Pully_belt calculations v6 (Autodesk Fusion 360 design; units mm, degrees)
Autodesk Fusion 360 part; units mm, degrees
(part 1 of 2)
ref_plane "WorkPlane1" through (0, 0, 0) normal (0, 0, 1) x (1, 0, 0)
sketch "Sketch2" plane through (0, 0, 0) normal (0, 0, 1) x (-1, 0, 0)
  line L0 (0, 0) -> (0, -17.9264) construction
  line L1 (0, 0) -> (0.956, -17.9285) construction
  arc A0 (-0.5778, -17.5255) -> (-0.6732, -17.788) centre (0.4, -18.0295) ccw
  arc A1 (0.6732, -17.788) -> (0.5778, -17.5255) centre (-0.4, -18.0295) ccw
  line L2 (0.6954, -17.9285) -> (-0.6954, -17.9285) construction
  arc A2 (0.5778, -17.5255) -> (-0.5778, -17.5255) centre (0, -17.8233) ccw
  line L3 (0, -17.8233) -> (0, -18.0295) construction
  line L4 (0.4, -18.0295) -> (-0.4, -18.0295) construction
  line L5 (0.8488, -17.9285) -> (0.956, -17.9285)
  line L6 (-0.8488, -17.9285) -> (-0.956, -17.9285)
  arc A3 (0.6732, -17.788) -> (0.8488, -17.9285) centre (0.8488, -17.7485) ccw
  arc A4 (-0.8488, -17.9285) -> (-0.6732, -17.788) centre (-0.8488, -17.7485) ccw
  line L7 (0.956, -17.9285) -> (0.6954, -17.9285) construction
  line L8 (-0.956, -17.9285) -> (-0.6954, -17.9285) construction
  line L9 (0, 0) -> (-0.956, -17.9285) construction
  circle A5 centre (0, 0) radius 17.954 construction
  arc A6 (2.4374, -17.3648) -> (1.2883, -17.4877) centre (1.8945, -17.7224) ccw
  arc A7 (2.5601, -17.6157) -> (2.4374, -17.3648) centre (1.5187, -17.9699) ccw
  arc A8 (2.5601, -17.6157) -> (2.7496, -17.7367) centre (2.7305, -17.5577) ccw
  line L10 (2.7496, -17.7367) -> (2.8563, -17.7253)
  arc A9 (1.0617, -17.9171) -> (1.2214, -17.7588) centre (1.0426, -17.7382) ccw
  arc A10 (1.2883, -17.4877) -> (1.2214, -17.7588) centre (2.3142, -17.8848) ccw
  line L11 (1.0617, -17.9171) -> (0.9551, -17.9285)
  arc A11 (4.2693, -17.0074) -> (3.1399, -17.2517) centre (3.7675, -17.4206) ccw
  arc A12 (4.418, -17.2438) -> (4.2693, -17.0074) centre (3.4202, -17.7066) ccw
  arc A13 (4.418, -17.2438) -> (4.6194, -17.3439) centre (4.5813, -17.168) ccw
  line L12 (4.6194, -17.3439) -> (4.7242, -17.3213)
  arc A14 (2.9602, -17.7028) -> (3.1021, -17.5283) centre (2.9221, -17.5268) ccw
  arc A15 (3.1399, -17.2517) -> (3.1021, -17.5283) centre (4.2021, -17.5375) ccw
  line L13 (2.9602, -17.7028) -> (2.8554, -17.7254)
  arc A16 (6.0529, -16.4572) -> (4.9558, -16.8202) centre (5.5979, -16.9214) ccw
  arc A17 (6.2259, -16.6765) -> (6.0529, -16.4572) centre (5.2829, -17.2428) ccw
  arc A18 (6.2259, -16.6765) -> (6.4367, -16.7547) centre (6.3802, -16.5838) ccw
  line L14 (6.4367, -16.7547) -> (6.5385, -16.721)
  arc A19 (4.8251, -17.2878) -> (4.9477, -17.0993) centre (4.7686, -17.1169) ccw
  arc A20 (4.9558, -16.8202) -> (4.9477, -17.0993) centre (6.0424, -16.9915) ccw
  line L15 (4.8251, -17.2878) -> (4.7233, -17.3215)
  arc A21 (7.7679, -15.7206) -> (6.7156, -16.1981) centre (7.3648, -16.2305) ccw
  arc A22 (7.9632, -15.9202) -> (7.7679, -15.7206) centre (7.0857, -16.5836) ccw
  arc A23 (7.9632, -15.9202) -> (8.1812, -15.9756) centre (8.1068, -15.8117) ccw
  line L16 (8.1812, -15.9756) -> (8.2788, -15.9313)
  arc A24 (6.6353, -16.677) -> (6.7372, -16.4765) centre (6.561, -16.5131) ccw
  arc A25 (6.7156, -16.1981) -> (6.7372, -16.4765) centre (7.8143, -16.253) ccw
  line L17 (6.6353, -16.677) -> (6.5377, -16.7213)
  arc A26 (9.3949, -14.8059) -> (8.3993, -15.3925) centre (9.0483, -15.3558) ccw
  arc A27 (9.6103, -14.9836) -> (9.3949, -14.8059) centre (8.8083, -15.7364) ccw
  arc A28 (9.6103, -14.9836) -> (9.8329, -15.0155) centre (9.7416, -14.8604) ccw
  line L18 (9.8329, -15.0155) -> (9.9253, -14.961)
  arc A29 (8.3704, -15.8772) -> (8.4504, -15.6671) centre (8.279, -15.7222) ccw
  arc A30 (8.3993, -15.3925) -> (8.4504, -15.6671) centre (9.4976, -15.3303) ccw
  line L19 (8.3704, -15.8772) -> (8.278, -15.9317)
  arc A31 (10.9155, -13.7234) -> (9.9879, -14.4125) centre (10.6293, -14.307) ccw
  arc A32 (11.1485, -13.8772) -> (10.9155, -13.7234) centre (10.4311, -14.711) ccw
  arc A33 (11.1485, -13.8772) -> (11.3733, -13.8852) centre (11.2659, -13.7407) ccw
  line L20 (11.3733, -13.8852) -> (11.4594, -13.8213)
  arc A34 (10.0106, -14.8976) -> (10.0678, -14.6801) centre (9.9033, -14.7531) ccw
  arc A35 (9.9879, -14.4125) -> (10.0678, -14.6801) centre (11.0733, -14.2339) ccw
  line L21 (10.0106, -14.8976) -> (9.9246, -14.9615)
  arc A36 (12.3123, -12.4854) -> (11.4633, -13.2692) centre (12.0898, -13.0961) ccw
  arc A37 (12.5604, -12.6135) -> (12.3123, -12.4854) centre (11.9357, -13.5189) ccw
  arc A38 (12.5604, -12.6135) -> (12.7848, -12.5977) centre (12.6627, -12.4654) ccw
  line L22 (12.7848, -12.5977) -> (12.8635, -12.5249)
  arc A39 (11.5374, -13.7491) -> (11.5712, -13.5268) centre (11.4153, -13.6169) ccw
  arc A40 (11.4633, -13.2692) -> (11.5712, -13.5268) centre (12.5235, -12.9763) ccw
  line L23 (11.5374, -13.7491) -> (11.4587, -13.8219)
  arc A41 (13.5697, -11.106) -> (12.8087, -11.9756) centre (13.4133, -11.7369) ccw
  arc A42 (13.83, -11.207) -> (13.5697, -11.106) centre (13.3051, -12.1736) ccw
  arc A43 (13.83, -11.207) -> (14.0514, -11.1673) centre (13.9159, -11.0488) ccw
  line L24 (14.0514, -11.1673) -> (14.122, -11.0867)
  arc A44 (12.9335, -12.4449) -> (12.9434, -12.2202) centre (12.7981, -12.3263) ccw
  arc A45 (12.8087, -11.9756) -> (12.9434, -12.2202) centre (13.8319, -11.5716) ccw
  line L25 (12.9335, -12.4449) -> (12.8629, -12.5256)
  arc A46 (14.6733, -9.6007) -> (14.0091, -10.5463) centre (14.5849, -10.2446) ccw
  arc A47 (14.9429, -9.6735) -> (14.6733, -9.6007) centre (14.5237, -10.6904) ccw
  arc A48 (14.9429, -9.6735) -> (15.1588, -9.6105) centre (15.0115, -9.507) ccw
  line L26 (15.1588, -9.6105) -> (15.2204, -9.5228)
  arc A49 (14.1831, -10.9996) -> (14.169, -10.7752) centre (14.0358, -10.8962) ccw
  arc A50 (14.0091, -10.5463) -> (14.169, -10.7752) centre (14.9835, -10.0358) ccw
  line L27 (14.1831, -10.9996) -> (14.1214, -11.0874)
  arc A51 (15.6107, -7.9866) -> (15.0507, -8.9974) centre (15.5912, -8.6363) ccw
  arc A52 (15.8865, -8.0303) -> (15.6107, -7.9866) centre (15.5777, -9.0861) ccw
  arc A53 (15.8865, -8.0303) -> (16.0944, -7.9448) centre (15.937, -7.8576) ccw
  line L28 (16.0944, -7.9448) -> (16.1464, -7.851)
  arc A54 (15.2719, -9.4297) -> (15.2341, -9.208) centre (15.1144, -9.3425) ccw
  arc A55 (15.0507, -8.9974) -> (15.2341, -9.208) centre (15.9653, -8.3863) ccw
  line L29 (15.2719, -9.4297) -> (15.2199, -9.5235)
  arc A56 (16.3712, -6.282) -> (15.9218, -7.3467) centre (16.4208, -6.9301) ccw
  arc A57 (16.65, -6.2962) -> (16.3712, -6.282) centre (16.4552, -7.3788) ccw
  arc A58 (16.65, -6.2962) -> (16.8477, -6.189) centre (16.6819, -6.1191) ccw
  line L30 (16.8477, -6.189) -> (16.8894, -6.0903)
  arc A59 (16.1877, -7.753) -> (16.1266, -7.5366) centre (16.0219, -7.683) ccw
  arc A60 (15.9218, -7.3467) -> (16.1266, -7.5366) centre (16.7663, -6.6418) ccw
  line L31 (16.1877, -7.753) -> (16.146, -7.8518)
  arc A61 (16.9461, -4.5063) -> (16.6125, -5.6127) centre (17.0644, -5.1455) ccw
  arc A62 (17.225, -4.4907) -> (16.9461, -4.5063) centre (17.1463, -5.5879) ccw
  arc A63 (17.225, -4.4907) -> (17.4102, -4.3632) centre (17.2378, -4.3112) ccw
  line L32 (17.4102, -4.3632) -> (17.4411, -4.2605)
  arc A64 (16.9201, -5.9884) -> (16.8363, -5.7798) centre (16.7478, -5.9365) ccw
  arc A65 (16.6125, -5.6127) -> (16.8363, -5.7798) centre (17.3773, -4.822) ccw
  line L33 (16.9201, -5.9884) -> (16.8891, -6.0911)
  arc A66 (17.3291, -2.6795) -> (17.115, -3.8151) centre (17.5147, -3.3025) ccw
  arc A67 (17.6047, -2.6344) -> (17.3291, -2.6795) centre (17.6432, -3.7337) ccw
  arc A68 (17.6047, -2.6344) -> (17.7753, -2.4879) centre (17.5984, -2.4545) ccw
  line L34 (17.7753, -2.4879) -> (17.7952, -2.3825)
  arc A69 (17.4608, -4.156) -> (17.3553, -3.9574) centre (17.2839, -4.1227) ccw
  arc A70 (17.115, -3.8151) -> (17.3553, -3.9574) centre (17.7914, -2.9476) ccw
  line L35 (17.4608, -4.156) -> (17.4409, -4.2614)
  arc A71 (17.5158, -0.8224) -> (17.4236, -1.9742) centre (17.7665, -1.4221) ccw
  arc A72 (17.785, -0.7482) -> (17.5158, -0.8224) centre (17.9401, -1.8372) ccw
  arc A73 (17.785, -0.7482) -> (17.939, -0.5844) centre (17.7596, -0.57) ccw
  line L36 (17.939, -0.5844) -> (17.9476, -0.4775)
  arc A74 (17.8036, -2.2765) -> (17.6776, -2.0903) centre (17.6242, -2.2622) ccw
  arc A75 (17.4236, -1.9742) -> (17.6776, -2.0903) centre (18.0039, -1.0398) ccw
  line L37 (17.8036, -2.2765) -> (17.795, -2.3834)
  arc A76 (17.504, 1.0441) -> (17.5347, -0.111) centre (17.817, 0.4745) ccw
  arc A77 (17.7638, 1.1465) -> (17.504, 1.0441) centre (18.0337, 0.0801) ccw
  arc A78 (17.7638, 1.1465) -> (17.8995, 1.3257) centre (17.7196, 1.3209) ccw
  line L38 (17.8995, 1.3257) -> (17.8967, 1.4329)
  arc A79 (17.9447, -0.3712) -> (17.7996, -0.1994) centre (17.7648, -0.376) ccw
  arc A80 (17.5347, -0.111) -> (17.7996, -0.1994) centre (18.0124, 0.8798) ccw
  line L39 (17.9447, -0.3712) -> (17.9476, -0.4784)
  arc A81 (17.2938, 2.8988) -> (17.4472, 1.7534) centre (17.6656, 2.3656) ccw
  arc A82 (17.5413, 3.0281) -> (17.2938, 2.8988) centre (17.9231, 1.9965) ccw
  arc A83 (17.5413, 3.0281) -> (17.6572, 3.2208) centre (17.4788, 3.1969) ccw
  line L40 (17.6572, 3.2208) -> (17.643, 3.3271)
  arc A84 (17.8825, 1.5383) -> (17.72, 1.6937) centre (17.7041, 1.5144) ccw
  arc A85 (17.4472, 1.7534) -> (17.72, 1.6937) centre (17.8169, 2.7894) ccw
  line L41 (17.8825, 1.5383) -> (17.8967, 1.432)
  arc A86 (16.8877, 4.7206) -> (17.162, 3.598) centre (17.3141, 4.23) ccw
  arc A87 (17.12, 4.8755) -> (16.8877, 4.7206) centre (17.6093, 3.8903) ccw
  arc A88 (17.12, 4.8755) -> (17.2148, 5.0794) centre (17.04, 5.0367) ccw
  line L42 (17.2148, 5.0794) -> (17.1894, 5.1836)
  arc A89 (17.6177, 3.4304) -> (17.4396, 3.5676) centre (17.4428, 3.3877) ccw
  arc A90 (17.162, 3.598) -> (17.4396, 3.5676) centre (17.4194, 4.6674) ccw
  line L43 (17.6177, 3.4304) -> (17.6431, 3.3262)
  arc A91 (16.2903, 6.4889) -> (16.6823, 5.4018) centre (16.7664, 6.0464) ccw
  arc A92 (16.5048, 6.6676) -> (16.2903, 6.4889) centre (17.096, 5.74) ccw
  arc A93 (16.5048, 6.6676) -> (16.5774, 6.8805) centre (16.4081, 6.8194) ccw
  line L44 (16.5774, 6.8805) -> (16.541, 6.9813)
  arc A94 (17.1533, 5.2836) -> (16.9615, 5.4011) centre (16.9839, 5.2225) ccw
  arc A95 (16.6823, 5.4018) -> (16.9615, 5.4011) centre (16.8246, 6.4926) ccw
  line L45 (17.1533, 5.2836) -> (17.1896, 5.1827)
  arc A96 (15.5083, 8.1837) -> (16.0136, 7.1444) centre (16.0287, 7.7943) ccw
  arc A97 (15.7026, 8.3842) -> (15.5083, 8.1837) centre (16.3891, 7.5247) ccw
  arc A98 (15.7026, 8.3842) -> (15.7521, 8.6036) centre (15.5902, 8.5249) ccw
  line L46 (15.7521, 8.6036) -> (15.7052, 8.7)
  arc A99 (16.4945, 7.0769) -> (16.2913, 7.1734) centre (16.3326, 6.9982) ccw
  arc A100 (16.0136, 7.1444) -> (16.2913, 7.1734) centre (16.0392, 8.2441) ccw
  line L47 (16.4945, 7.0769) -> (16.5414, 6.9805)
  arc A101 (14.5505, 9.7857) -> (15.1635, 8.8061) centre (15.1094, 9.4539) ccw
  arc A102 (14.7224, 10.0058) -> (14.5505, 9.7857) centre (15.4964, 9.2241) ccw
  arc A103 (14.7224, 10.0058) -> (14.7484, 10.2292) centre (14.5958, 10.1337) ccw
  line L48 (14.7484, 10.2292) -> (14.6915, 10.3201)
  arc A104 (15.6488, 8.7901) -> (15.4366, 8.8645) centre (15.4962, 8.6946) ccw
  arc A105 (15.1635, 8.8061) -> (15.4366, 8.8645) centre (15.072, 9.9023) ccw
  line L49 (15.6488, 8.7901) -> (15.7057, 8.6992)
  arc A106 (13.428, 11.2769) -> (14.1415, 10.368) centre (14.019, 11.0063) ccw
  arc A107 (13.5755, 11.514) -> (13.428, 11.2769) centre (14.4281, 10.819) ccw
  arc A108 (13.5755, 11.514) -> (13.5775, 11.7389) centre (13.436, 11.6277) ccw
  line L50 (13.5775, 11.7389) -> (13.5113, 11.8232)
  arc A109 (14.6258, 10.4037) -> (14.4069, 10.455) centre (14.4842, 10.2925) ccw
  arc A110 (14.1415, 10.368) -> (14.4069, 10.455) centre (13.9341, 11.4483) ccw
  line L51 (14.6258, 10.4037) -> (14.692, 10.3193)
  arc A111 (12.1532, 12.6403) -> (12.9594, 11.8124) centre (12.7696, 12.4341) ccw
  arc A112 (12.2747, 12.8918) -> (12.1532, 12.6403) centre (13.1964, 12.2914) ccw
  arc A113 (12.2747, 12.8918) -> (12.2528, 13.1156) centre (12.1239, 12.99) ccw
  line L52 (12.2528, 13.1156) -> (12.178, 13.1924)
  arc A114 (13.4371, 11.8994) -> (13.214, 11.9272) centre (13.3082, 11.7738) ccw
  arc A115 (12.9594, 11.8124) -> (13.214, 11.9272) centre (12.6383, 12.8645) ccw
  line L53 (13.4371, 11.8994) -> (13.5119, 11.8225)
  arc A116 (10.7408, 13.8605) -> (11.6304, 13.123) centre (11.3756, 13.721) ccw
  arc A117 (10.8349, 14.1234) -> (10.7408, 13.8605) centre (11.8151, 13.6244) ccw
  arc A118 (10.8349, 14.1234) -> (10.7893, 14.3437) centre (10.6744, 14.2051) ccw
  line L54 (10.7893, 14.3437) -> (10.7068, 14.4121)
  arc A119 (12.0962, 13.2602) -> (11.8713, 13.2642) centre (11.9813, 13.1217) ccw
  arc A120 (11.6304, 13.123) -> (11.8713, 13.2642) centre (11.1993, 14.135) ccw
  line L55 (12.0962, 13.2602) -> (12.1787, 13.1918)
  arc A121 (9.2067, 14.9237) -> (10.1696, 14.2849) centre (9.8527, 14.8524) ccw
  arc A122 (9.2722, 15.1951) -> (9.2067, 14.9237) centre (10.3, 14.8031) ccw
  arc A123 (9.2722, 15.1951) -> (9.2036, 15.4093) centre (9.1041, 15.2593) ccw
  line L56 (9.2036, 15.4093) -> (9.1142, 15.4685)
  arc A124 (10.6182, 14.4708) -> (10.3942, 14.4509) centre (10.5187, 14.3209) ccw
  arc A125 (10.1696, 14.2849) -> (10.3942, 14.4509) centre (9.6334, 15.2453) ccw
  line L57 (10.6182, 14.4708) -> (10.7075, 14.4116)
  arc A126 (7.5682, 15.8177) -> (8.5936, 15.2849) centre (8.2182, 15.8156) ccw
  arc A127 (7.6046, 16.0946) -> (7.5682, 15.8177) centre (8.6682, 15.8141) ccw
  arc A128 (7.6046, 16.0946) -> (7.5135, 16.3002) centre (7.4305, 16.1405) ccw
  line L58 (7.5135, 16.3002) -> (7.4184, 16.3497)
  arc A129 (9.0199, 15.5175) -> (8.7992, 15.4738) centre (8.9369, 15.3578) ccw
  arc A130 (8.5936, 15.2849) -> (8.7992, 15.4738) centre (7.9583, 16.1829) ccw
  line L59 (9.0199, 15.5175) -> (9.115, 15.4681)
  arc A131 (5.844, 16.5326) -> (6.9202, 16.1118) centre (6.4906, 16.5995) ccw
  arc A132 (5.8507, 16.8117) -> (5.844, 16.5326) centre (6.9382, 16.6458) ccw
  arc A133 (5.8507, 16.8117) -> (5.7384, 17.0065) centre (5.6728, 16.8389) ccw
  line L60 (5.7384, 17.0065) -> (5.6385, 17.0456)
  arc A134 (7.3193, 16.3884) -> (7.1046, 16.3215) centre (7.2538, 16.2207) ccw
  arc A135 (6.9202, 16.1118) -> (7.1046, 16.3215) centre (6.1931, 16.9372) ccw
  line L61 (7.3193, 16.3884) -> (7.4192, 16.3493)
  arc A136 (4.0536, 17.0601) -> (5.1684, 16.7561) centre (4.6894, 17.1954) ccw
  arc A137 (4.0306, 17.3384) -> (4.0536, 17.0601) centre (5.1295, 17.289) ccw
  arc A138 (4.0306, 17.3384) -> (3.8982, 17.5201) centre (3.8508, 17.3465) ccw
  line L62 (3.8982, 17.5201) -> (3.7947, 17.5483)
  arc A139 (5.5359, 17.0735) -> (5.3295, 16.9842) centre (5.4885, 16.8998) ccw
  arc A140 (5.1684, 16.7561) -> (5.3295, 16.9842) centre (4.3577, 17.4995) ccw
  line L63 (5.5359, 17.0735) -> (5.6393, 17.0453)
  arc A141 (2.2173, 17.3943) -> (3.3581, 17.2105) centre (2.835, 17.5964) ccw
  arc A142 (2.1648, 17.6686) -> (2.2173, 17.3943) centre (3.2627, 17.7363) ccw
  arc A143 (2.1648, 17.6686) -> (2.0138, 17.8352) centre (1.9852, 17.6575) ccw
  line L64 (2.0138, 17.8352) -> (1.9079, 17.8523)
  arc A144 (3.6897, 17.5652) -> (3.494, 17.4544) centre (3.6611, 17.3875) ccw
  arc A145 (3.3581, 17.2105) -> (3.494, 17.4544) centre (2.4729, 17.8636) ccw
  line L65 (3.6897, 17.5652) -> (3.7956, 17.5482)
  arc A146 (0.3558, 17.5315) -> (1.5097, 17.47) centre (0.9486, 17.7981) ccw
  arc A147 (0.2745, 17.7986) -> (0.3558, 17.5315) centre (1.359, 17.9826) ccw
  arc A148 (0.2745, 17.7986) -> (0.1066, 17.9482) centre (0.097, 17.7685) ccw
  line L66 (0.1066, 17.9482) -> (-0.0005, 17.954)
  arc A149 (1.8018, 17.8579) -> (1.6189, 17.727) centre (1.7922, 17.6782) ccw
  arc A150 (1.5097, 17.47) -> (1.6189, 17.727) centre (0.5601, 18.0252) ccw
  line L67 (1.8018, 17.8579) -> (1.9088, 17.8522)
  arc A151 (-1.5097, 17.47) -> (-0.3558, 17.5315) centre (-0.9486, 17.7981) ccw
  arc A152 (-1.6189, 17.727) -> (-1.5097, 17.47) centre (-0.5601, 18.0252) ccw
  arc A153 (-1.6189, 17.727) -> (-1.8018, 17.8579) centre (-1.7922, 17.6782) ccw
  line L68 (-1.8018, 17.8579) -> (-1.9088, 17.8522)
  arc A154 (-0.1066, 17.9482) -> (-0.2745, 17.7986) centre (-0.097, 17.7685) ccw
  arc A155 (-0.3558, 17.5315) -> (-0.2745, 17.7986) centre (-1.359, 17.9826) ccw
  line L69 (-0.1066, 17.9482) -> (0.0005, 17.954)
  arc A156 (-3.3581, 17.2105) -> (-2.2173, 17.3943) centre (-2.835, 17.5964) ccw
  arc A157 (-3.494, 17.4544) -> (-3.3581, 17.2105) centre (-2.4729, 17.8636) ccw
  arc A158 (-3.494, 17.4544) -> (-3.6897, 17.5652) centre (-3.6611, 17.3875) ccw
  line L70 (-3.6897, 17.5652) -> (-3.7956, 17.5482)
  arc A159 (-2.0138, 17.8352) -> (-2.1648, 17.6686) centre (-1.9852, 17.6575) ccw
  arc A160 (-2.2173, 17.3943) -> (-2.1648, 17.6686) centre (-3.2627, 17.7363) ccw
  line L71 (-2.0138, 17.8352) -> (-1.9079, 17.8523)
  arc A161 (-5.1684, 16.7561) -> (-4.0536, 17.0601) centre (-4.6894, 17.1954) ccw
  arc A162 (-5.3295, 16.9842) -> (-5.1684, 16.7561) centre (-4.3577, 17.4995) ccw
  arc A163 (-5.3295, 16.9842) -> (-5.5359, 17.0735) centre (-5.4885, 16.8998) ccw
  line L72 (-5.5359, 17.0735) -> (-5.6393, 17.0453)
  arc A164 (-3.8982, 17.5201) -> (-4.0306, 17.3384) centre (-3.8508, 17.3465) ccw
  arc A165 (-4.0536, 17.0601) -> (-4.0306, 17.3384) centre (-5.1295, 17.289) ccw
  line L73 (-3.8982, 17.5201) -> (-3.7947, 17.5483)
  arc A166 (-6.9202, 16.1118) -> (-5.844, 16.5326) centre (-6.4906, 16.5995) ccw
  arc A167 (-7.1046, 16.3215) -> (-6.9202, 16.1118) centre (-6.1931, 16.9372) ccw
  arc A168 (-7.1046, 16.3215) -> (-7.3193, 16.3884) centre (-7.2538, 16.2207) ccw
  line L74 (-7.3193, 16.3884) -> (-7.4192, 16.3493)
  arc A169 (-5.7384, 17.0065) -> (-5.8507, 16.8117) centre (-5.6728, 16.8389) ccw
  arc A170 (-5.844, 16.5326) -> (-5.8507, 16.8117) centre (-6.9382, 16.6458) ccw
  line L75 (-5.7384, 17.0065) -> (-5.6385, 17.0456)
  arc A171 (-8.5936, 15.2849) -> (-7.5682, 15.8177) centre (-8.2182, 15.8156) ccw
  arc A172 (-8.7992, 15.4738) -> (-8.5936, 15.2849) centre (-7.9583, 16.1829) ccw
  arc A173 (-8.7992, 15.4738) -> (-9.0199, 15.5175) centre (-8.9369, 15.3578) ccw
  line L76 (-9.0199, 15.5175) -> (-9.115, 15.4681)
  arc A174 (-7.5135, 16.3002) -> (-7.6046, 16.0946) centre (-7.4305, 16.1405) ccw
  arc A175 (-7.5682, 15.8177) -> (-7.6046, 16.0946) centre (-8.6682, 15.8141) ccw
  line L77 (-7.5135, 16.3002) -> (-7.4184, 16.3497)
  arc A176 (-10.1696, 14.2849) -> (-9.2067, 14.9237) centre (-9.8527, 14.8524) ccw
  arc A177 (-10.3942, 14.4509) -> (-10.1696, 14.2849) centre (-9.6334, 15.2453) ccw
  arc A178 (-10.3942, 14.4509) -> (-10.6182, 14.4708) centre (-10.5187, 14.3209) ccw
  line L78 (-10.6182, 14.4708) -> (-10.7075, 14.4116)
  arc A179 (-9.2036, 15.4093) -> (-9.2722, 15.1951) centre (-9.1041, 15.2593) ccw
  arc A180 (-9.2067, 14.9237) -> (-9.2722, 15.1951) centre (-10.3, 14.8031) ccw
  line L79 (-9.2036, 15.4093) -> (-9.1142, 15.4685)
  arc A181 (-11.6304, 13.123) -> (-10.7408, 13.8605) centre (-11.3756, 13.721) ccw
  arc A182 (-11.8713, 13.2642) -> (-11.6304, 13.123) centre (-11.1993, 14.135) ccw
  arc A183 (-11.8713, 13.2642) -> (-12.0962, 13.2602) centre (-11.9813, 13.1217) ccw
  line L80 (-12.0962, 13.2602) -> (-12.1787, 13.1918)
  arc A184 (-10.7893, 14.3437) -> (-10.8349, 14.1234) centre (-10.6744, 14.2051) ccw
  arc A185 (-10.7408, 13.8605) -> (-10.8349, 14.1234) centre (-11.8151, 13.6244) ccw
  line L81 (-10.7893, 14.3437) -> (-10.7068, 14.4121)
  arc A186 (-12.9594, 11.8124) -> (-12.1532, 12.6403) centre (-12.7696, 12.4341) ccw
  arc A187 (-13.214, 11.9272) -> (-12.9594, 11.8124) centre (-12.6383, 12.8645) ccw
  arc A188 (-13.214, 11.9272) -> (-13.4371, 11.8994) centre (-13.3082, 11.7738) ccw
  line L82 (-13.4371, 11.8994) -> (-13.5119, 11.8225)
  arc A189 (-12.2528, 13.1156) -> (-12.2747, 12.8918) centre (-12.1239, 12.99) ccw
  arc A190 (-12.1532, 12.6403) -> (-12.2747, 12.8918) centre (-13.1964, 12.2914) ccw
  line L83 (-12.2528, 13.1156) -> (-12.178, 13.1924)
  arc A191 (-14.1415, 10.368) -> (-13.428, 11.2769) centre (-14.019, 11.0063) ccw
  arc A192 (-14.4069, 10.455) -> (-14.1415, 10.368) centre (-13.9341, 11.4483) ccw
  arc A193 (-14.4069, 10.455) -> (-14.6258, 10.4037) centre (-14.4842, 10.2925) ccw
  line L84 (-14.6258, 10.4037) -> (-14.692, 10.3193)
  arc A194 (-13.5775, 11.7389) -> (-13.5755, 11.514) centre (-13.436, 11.6277) ccw
  arc A195 (-13.428, 11.2769) -> (-13.5755, 11.514) centre (-14.4281, 10.819) ccw
  line L85 (-13.5775, 11.7389) -> (-13.5113, 11.8232)
  arc A196 (-15.1635, 8.8061) -> (-14.5505, 9.7857) centre (-15.1094, 9.4539) ccw
  arc A197 (-15.4366, 8.8645) -> (-15.1635, 8.8061) centre (-15.072, 9.9023) ccw
  arc A198 (-15.4366, 8.8645) -> (-15.6488, 8.7901) centre (-15.4962, 8.6946) ccw
  line L86 (-15.6488, 8.7901) -> (-15.7057, 8.6992)
  arc A199 (-14.7484, 10.2292) -> (-14.7224, 10.0058) centre (-14.5958, 10.1337) ccw
  arc A200 (-14.5505, 9.7857) -> (-14.7224, 10.0058) centre (-15.4964, 9.2241) ccw
  line L87 (-14.7484, 10.2292) -> (-14.6915, 10.3201)
  arc A201 (-16.0136, 7.1444) -> (-15.5083, 8.1837) centre (-16.0287, 7.7943) ccw
  arc A202 (-16.2913, 7.1734) -> (-16.0136, 7.1444) centre (-16.0392, 8.2441) ccw
  arc A203 (-16.2913, 7.1734) -> (-16.4945, 7.0769) centre (-16.3326, 6.9982) ccw
  line L88 (-16.4945, 7.0769) -> (-16.5414, 6.9805)
  arc A204 (-15.7521, 8.6036) -> (-15.7026, 8.3842) centre (-15.5902, 8.5249) ccw
  arc A205 (-15.5083, 8.1837) -> (-15.7026, 8.3842) centre (-16.3891, 7.5247) ccw
  line L89 (-15.7521, 8.6036) -> (-15.7052, 8.7)
  arc A206 (-16.6823, 5.4018) -> (-16.2903, 6.4889) centre (-16.7664, 6.0464) ccw
  arc A207 (-16.9615, 5.4011) -> (-16.6823, 5.4018) centre (-16.8246, 6.4926) ccw
  arc A208 (-16.9615, 5.4011) -> (-17.1533, 5.2836) centre (-16.9839, 5.2225) ccw
  line L90 (-17.1533, 5.2836) -> (-17.1896, 5.1827)
  arc A209 (-16.5774, 6.8805) -> (-16.5048, 6.6676) centre (-16.4081, 6.8194) ccw
  arc A210 (-16.2903, 6.4889) -> (-16.5048, 6.6676) centre (-17.096, 5.74) ccw
  line L91 (-16.5774, 6.8805) -> (-16.541, 6.9813)
  arc A211 (-17.162, 3.598) -> (-16.8877, 4.7206) centre (-17.3141, 4.23) ccw
  arc A212 (-17.4396, 3.5676) -> (-17.162, 3.598) centre (-17.4194, 4.6674) ccw
  arc A213 (-17.4396, 3.5676) -> (-17.6177, 3.4304) centre (-17.4428, 3.3877) ccw
  line L92 (-17.6177, 3.4304) -> (-17.6431, 3.3262)
  arc A214 (-17.2148, 5.0794) -> (-17.12, 4.8755) centre (-17.04, 5.0367) ccw
  arc A215 (-16.8877, 4.7206) -> (-17.12, 4.8755) centre (-17.6093, 3.8903) ccw
  line L93 (-17.2148, 5.0794) -> (-17.1894, 5.1836)
  arc A216 (-17.4472, 1.7534) -> (-17.2938, 2.8988) centre (-17.6656, 2.3656) ccw
  arc A217 (-17.72, 1.6937) -> (-17.4472, 1.7534) centre (-17.8169, 2.7894) ccw
  arc A218 (-17.72, 1.6937) -> (-17.8825, 1.5383) centre (-17.7041, 1.5144) ccw
  line L94 (-17.8825, 1.5383) -> (-17.8967, 1.432)
  arc A219 (-17.6572, 3.2208) -> (-17.5413, 3.0281) centre (-17.4788, 3.1969) ccw
  arc A220 (-17.2938, 2.8988) -> (-17.5413, 3.0281) centre (-17.9231, 1.9965) ccw
  line L95 (-17.6572, 3.2208) -> (-17.643, 3.3271)
  arc A221 (-17.5347, -0.111) -> (-17.504, 1.0441) centre (-17.817, 0.4745) ccw
  arc A222 (-17.7996, -0.1994) -> (-17.5347, -0.111) centre (-18.0124, 0.8798) ccw
  arc A223 (-17.7996, -0.1994) -> (-17.9447, -0.3712) centre (-17.7648, -0.376) ccw
  line L96 (-17.9447, -0.3712) -> (-17.9476, -0.4784)
  arc A224 (-17.8995, 1.3257) -> (-17.7638, 1.1465) centre (-17.7196, 1.3209) ccw
  arc A225 (-17.504, 1.0441) -> (-17.7638, 1.1465) centre (-18.0337, 0.0801) ccw
  line L97 (-17.8995, 1.3257) -> (-17.8967, 1.4329)
  arc A226 (-17.4236, -1.9742) -> (-17.5158, -0.8224) centre (-17.7665, -1.4221) ccw
  arc A227 (-17.6776, -2.0903) -> (-17.4236, -1.9742) centre (-18.0039, -1.0398) ccw
  arc A228 (-17.6776, -2.0903) -> (-17.8036, -2.2765) centre (-17.6242, -2.2622) ccw
  line L98 (-17.8036, -2.2765) -> (-17.795, -2.3834)
  arc A229 (-17.939, -0.5844) -> (-17.785, -0.7482) centre (-17.7596, -0.57) ccw
  arc A230 (-17.5158, -0.8224) -> (-17.785, -0.7482) centre (-17.9401, -1.8372) ccw
  line L99 (-17.939, -0.5844) -> (-17.9476, -0.4775)
  arc A231 (-17.115, -3.8151) -> (-17.3291, -2.6795) centre (-17.5147, -3.3025) ccw
  arc A232 (-17.3553, -3.9574) -> (-17.115, -3.8151) centre (-17.7914, -2.9476) ccw
  arc A233 (-17.3553, -3.9574) -> (-17.4608, -4.156) centre (-17.2839, -4.1227) ccw
  line L100 (-17.4608, -4.156) -> (-17.4409, -4.2614)
  arc A234 (-17.7753, -2.4879) -> (-17.6047, -2.6344) centre (-17.5984, -2.4545) ccw
  arc A235 (-17.3291, -2.6795) -> (-17.6047, -2.6344) centre (-17.6432, -3.7337) ccw
  line L101 (-17.7753, -2.4879) -> (-17.7952, -2.3825)
  arc A236 (-16.6125, -5.6127) -> (-16.9461, -4.5063) centre (-17.0644, -5.1455) ccw
  arc A237 (-16.8363, -5.7798) -> (-16.6125, -5.6127) centre (-17.3773, -4.822) ccw
  arc A238 (-16.8363, -5.7798) -> (-16.9201, -5.9884) centre (-16.7478, -5.9365) ccw
  line L102 (-16.9201, -5.9884) -> (-16.8891, -6.0911)
  arc A239 (-17.4102, -4.3632) -> (-17.225, -4.4907) centre (-17.2378, -4.3112) ccw
  arc A240 (-16.9461, -4.5063) -> (-17.225, -4.4907) centre (-17.1463, -5.5879) ccw
  line L103 (-17.4102, -4.3632) -> (-17.4411, -4.2605)
  arc A241 (-15.9218, -7.3467) -> (-16.3712, -6.282) centre (-16.4208, -6.9301) ccw
  arc A242 (-16.1266, -7.5366) -> (-15.9218, -7.3467) centre (-16.7663, -6.6418) ccw
  arc A243 (-16.1266, -7.5366) -> (-16.1877, -7.753) centre (-16.0219, -7.683) ccw
  line L104 (-16.1877, -7.753) -> (-16.146, -7.8518)
  arc A244 (-16.8477, -6.189) -> (-16.65, -6.2962) centre (-16.6819, -6.1191) ccw
  arc A245 (-16.3712, -6.282) -> (-16.65, -6.2962) centre (-16.4552, -7.3788) ccw
  line L105 (-16.8477, -6.189) -> (-16.8894, -6.0903)
  arc A246 (-15.0507, -8.9974) -> (-15.6107, -7.9866) centre (-15.5912, -8.6363) ccw
  arc A247 (-15.2341, -9.208) -> (-15.0507, -8.9974) centre (-15.9653, -8.3863) ccw
  arc A248 (-15.2341, -9.208) -> (-15.2719, -9.4297) centre (-15.1144, -9.3425) ccw
  line L106 (-15.2719, -9.4297) -> (-15.2199, -9.5235)
  arc A249 (-16.0944, -7.9448) -> (-15.8865, -8.0303) centre (-15.937, -7.8576) ccw
  arc A250 (-15.6107, -7.9866) -> (-15.8865, -8.0303) centre (-15.5777, -9.0861) ccw
  line L107 (-16.0944, -7.9448) -> (-16.1464, -7.851)
  arc A251 (-14.0091, -10.5463) -> (-14.6733, -9.6007) centre (-14.5849, -10.2446) ccw
  arc A252 (-14.169, -10.7752) -> (-14.0091, -10.5463) centre (-14.9835, -10.0358) ccw
  arc A253 (-14.169, -10.7752) -> (-14.1831, -10.9996) centre (-14.0358, -10.8962) ccw
  line L108 (-14.1831, -10.9996) -> (-14.1214, -11.0874)
  arc A254 (-15.1588, -9.6105) -> (-14.9429, -9.6735) centre (-15.0115, -9.507) ccw
  arc A255 (-14.6733, -9.6007) -> (-14.9429, -9.6735) centre (-14.5237, -10.6904) ccw
  line L109 (-15.1588, -9.6105) -> (-15.2204, -9.5228)
  arc A256 (-12.8087, -11.9756) -> (-13.5697, -11.106) centre (-13.4133, -11.7369) ccw
  arc A257 (-12.9434, -12.2202) -> (-12.8087, -11.9756) centre (-13.8319, -11.5716) ccw
  arc A258 (-12.9434, -12.2202) -> (-12.9335, -12.4449) centre (-12.7981, -12.3263) ccw
  line L110 (-12.9335, -12.4449) -> (-12.8629, -12.5256)
  arc A259 (-14.0514, -11.1673) -> (-13.83, -11.207) centre (-13.9159, -11.0488) ccw
  arc A260 (-13.5697, -11.106) -> (-13.83, -11.207) centre (-13.3051, -12.1736) ccw
  line L111 (-14.0514, -11.1673) -> (-14.122, -11.0867)
  arc A261 (-11.4633, -13.2692) -> (-12.3123, -12.4854) centre (-12.0898, -13.0961) ccw
  arc A262 (-11.5712, -13.5268) -> (-11.4633, -13.2692) centre (-12.5235, -12.9763) ccw
  arc A263 (-11.5712, -13.5268) -> (-11.5374, -13.7491) centre (-11.4153, -13.6169) ccw
  line L112 (-11.5374, -13.7491) -> (-11.4587, -13.8219)
  arc A264 (-12.7848, -12.5976) -> (-12.5604, -12.6135) centre (-12.6627, -12.4654) ccw
  arc A265 (-12.3123, -12.4854) -> (-12.5604, -12.6135) centre (-11.9357, -13.5189) ccw
  line L113 (-12.7848, -12.5976) -> (-12.8635, -12.5249)
  arc A266 (-9.9879, -14.4125) -> (-10.9155, -13.7234) centre (-10.6293, -14.307) ccw
  arc A267 (-10.0678, -14.6801) -> (-9.9879, -14.4125) centre (-11.0733, -14.2339) ccw
  arc A268 (-10.0678, -14.6801) -> (-10.0106, -14.8976) centre (-9.9033, -14.7531) ccw
  line L114 (-10.0106, -14.8976) -> (-9.9246, -14.9615)
  arc A269 (-11.3733, -13.8852) -> (-11.1485, -13.8772) centre (-11.2659, -13.7407) ccw
  arc A270 (-10.9155, -13.7234) -> (-11.1485, -13.8772) centre (-10.4311, -14.711) ccw
  line L115 (-11.3733, -13.8852) -> (-11.4594, -13.8213)
  arc A271 (-8.3993, -15.3925) -> (-9.3949, -14.8059) centre (-9.0483, -15.3558) ccw
  arc A272 (-8.4504, -15.6671) -> (-8.3993, -15.3925) centre (-9.4976, -15.3303) ccw
  arc A273 (-8.4504, -15.6671) -> (-8.3704, -15.8772) centre (-8.279, -15.7222) ccw
  line L116 (-8.3704, -15.8772) -> (-8.278, -15.9317)
  arc A274 (-9.8329, -15.0155) -> (-9.6103, -14.9836) centre (-9.7416, -14.8604) ccw
  arc A275 (-9.3949, -14.8059) -> (-9.6103, -14.9836) centre (-8.8083, -15.7364) ccw
  line L117 (-9.8329, -15.0155) -> (-9.9253, -14.961)
  arc A276 (-6.7156, -16.1981) -> (-7.7679, -15.7206) centre (-7.3648, -16.2305) ccw
  arc A277 (-6.7372, -16.4765) -> (-6.7156, -16.1981) centre (-7.8143, -16.253) ccw
  arc A278 (-6.7372, -16.4765) -> (-6.6353, -16.677) centre (-6.561, -16.5131) ccw
  line L118 (-6.6353, -16.677) -> (-6.5377, -16.7213)
  arc A279 (-8.1812, -15.9756) -> (-7.9632, -15.9202) centre (-8.1068, -15.8117) ccw
  arc A280 (-7.7679, -15.7206) -> (-7.9632, -15.9202) centre (-7.0857, -16.5836) ccw
  line L119 (-8.1812, -15.9756) -> (-8.2788, -15.9313)
  arc A281 (-4.9558, -16.8202) -> (-6.0529, -16.4572) centre (-5.5979, -16.9214) ccw
  arc A282 (-4.9477, -17.0993) -> (-4.9558, -16.8202) centre (-6.0424, -16.9915) ccw
  arc A283 (-4.9477, -17.0993) -> (-4.8251, -17.2878) centre (-4.7686, -17.1169) ccw
  line L120 (-4.8251, -17.2878) -> (-4.7233, -17.3215)
  arc A284 (-6.4367, -16.7547) -> (-6.2259, -16.6765) centre (-6.3802, -16.5838) ccw
  arc A285 (-6.0529, -16.4572) -> (-6.2259, -16.6765) centre (-5.2829, -17.2428) ccw
  line L121 (-6.4367, -16.7547) -> (-6.5385, -16.721)
  arc A286 (-3.1399, -17.2517) -> (-4.2693, -17.0074) centre (-3.7675, -17.4206) ccw
  arc A287 (-3.1021, -17.5283) -> (-3.1399, -17.2517) centre (-4.2021, -17.5375) ccw
  arc A288 (-3.1021, -17.5283) -> (-2.9602, -17.7028) centre (-2.9221, -17.5268) ccw
  line L122 (-2.9602, -17.7028) -> (-2.8554, -17.7254)
  arc A289 (-4.6194, -17.3439) -> (-4.418, -17.2438) centre (-4.5813, -17.168) ccw
  arc A290 (-4.2693, -17.0074) -> (-4.418, -17.2438) centre (-3.4202, -17.7066) ccw
  line L123 (-4.6194, -17.3439) -> (-4.7242, -17.3213)
  arc A291 (-1.2883, -17.4877) -> (-2.4374, -17.3648) centre (-1.8945, -17.7224) ccw
  arc A292 (-1.2214, -17.7588) -> (-1.2883, -17.4877) centre (-2.3142, -17.8848) ccw
  arc A293 (-1.2214, -17.7588) -> (-1.0617, -17.9171) centre (-1.0426, -17.7382) ccw
  line L124 (-1.0617, -17.9171) -> (-0.9551, -17.9285)
  arc A294 (-2.7496, -17.7367) -> (-2.5601, -17.6157) centre (-2.7305, -17.5577) ccw
  arc A295 (-2.4374, -17.3648) -> (-2.5601, -17.6157) centre (-1.5187, -17.9699) ccw
  line L125 (-2.7496, -17.7367) -> (-2.8563, -17.7253)
  dimension "d14" = 1.1
  dimension "d18" = 1.1
  dimension "d19" = 0.65
  dimension "d22" = 0.8
  dimension "d25" = 0.18
  dimension "d26" = 0.18
  dimension "d27" = 0.101
  dimension "d28" = 1.912
  dimension "d29" = 0.2062
  dimension "d31" = 35.9079
  dimension "d65" = 360
  constraint vertical L0
  constraint coincident L0 A2.centre
  constraint coincident L0.start L1.start
  constraint tangent A0 A2
  constraint tangent A1 A2
  constraint coincident A2.centre L3.start
  constraint coincident A0.centre L4.start
  constraint coincident A1.centre L4.end
  constraint horizontal L4
  constraint midpoint L3.end L4
  constraint coincident L1 L5.end
  constraint parallel L2 L5
  constraint parallel L2 L6
  constraint coincident L1.end L5.end
  constraint coincident L2.start L5
  constraint coincident A1 L2.start
  constraint tangent L5 A3
  constraint tangent A1 A3
  constraint coincident L2.end L6
  constraint coincident A0 L2.end
  constraint tangent A0 A4
  constraint tangent L6 A4
  constraint equal L5 L6
  constraint parallel L2 L8
  constraint equal L7 L8
  constraint midpoint L0.end L3
  constraint coincident L1.end A5
  measures "d14" radius of A1
  measures "d18" radius of A0
  measures "d19" radius of A2
  measures "d22" distance of A0.centre A1.centre
  measures "d25" radius of A3
  measures "d26" radius of A4
  measures "d27" distance of L2 L4
  measures "d28" distance of L1.end L6.end
  measures "d29" distance of A2.centre L4
  measures "d31" diameter of A5
extrude "Extrude2" add sketch "Sketch2" along normal blind 7
sketch "Sketch11" plane through (0, 0, 7) normal (0, 0, 1) x (-1, 0, 0)
  arc A0 (-1.2214, -17.7588) -> (-1.0617, -17.9171) centre (-1.0426, -17.7382) ccw
  line L0 (-1.0617, -17.9171) -> (-0.9555, -17.9285)
  line L1 (-0.9555, -17.9285) -> (-0.8488, -17.9285)
  arc A1 (-0.8488, -17.9285) -> (-0.6732, -17.788) centre (-0.8488, -17.7485) ccw
  arc A2 (-0.5778, -17.5255) -> (-0.6732, -17.788) centre (0.4, -18.0295) ccw
  arc A3 (0.5778, -17.5255) -> (-0.5778, -17.5255) centre (0, -17.8233) ccw
  arc A4 (0.6732, -17.788) -> (0.5778, -17.5255) centre (-0.4, -18.0295) ccw
  arc A5 (0.6732, -17.788) -> (0.8488, -17.9285) centre (0.8488, -17.7485) ccw
  line L2 (0.8488, -17.9285) -> (0.9555, -17.9285)
  line L3 (0.9555, -17.9285) -> (1.0617, -17.9171)
  arc A6 (1.0617, -17.9171) -> (1.2214, -17.7588) centre (1.0426, -17.7382) ccw
  arc A7 (1.2883, -17.4877) -> (1.2214, -17.7588) centre (2.3142, -17.8848) ccw
  arc A8 (2.4374, -17.3648) -> (1.2883, -17.4877) centre (1.8945, -17.7224) ccw
  arc A9 (2.5601, -17.6157) -> (2.4374, -17.3648) centre (1.5187, -17.9699) ccw
  arc A10 (2.5601, -17.6157) -> (2.7496, -17.7367) centre (2.7305, -17.5577) ccw
  line L4 (2.7496, -17.7367) -> (2.8558, -17.7253)
  line L5 (2.8558, -17.7253) -> (2.9602, -17.7028)
  arc A11 (2.9602, -17.7028) -> (3.1021, -17.5283) centre (2.9221, -17.5268) ccw
  arc A12 (3.1399, -17.2517) -> (3.1021, -17.5283) centre (4.2021, -17.5375) ccw
  arc A13 (4.2693, -17.0074) -> (3.1399, -17.2517) centre (3.7675, -17.4206) ccw
  arc A14 (4.418, -17.2438) -> (4.2693, -17.0074) centre (3.4202, -17.7066) ccw
  arc A15 (4.418, -17.2438) -> (4.6194, -17.3439) centre (4.5813, -17.168) ccw
  line L6 (4.6194, -17.3439) -> (4.7237, -17.3214)
  line L7 (4.7237, -17.3214) -> (4.8251, -17.2878)
  arc A16 (4.8251, -17.2878) -> (4.9477, -17.0993) centre (4.7686, -17.1169) ccw
  arc A17 (4.9558, -16.8202) -> (4.9477, -17.0993) centre (6.0424, -16.9915) ccw
  arc A18 (6.0529, -16.4572) -> (4.9558, -16.8202) centre (5.5979, -16.9214) ccw
  arc A19 (6.2259, -16.6765) -> (6.0529, -16.4572) centre (5.2829, -17.2428) ccw
  arc A20 (6.2259, -16.6765) -> (6.4367, -16.7547) centre (6.3802, -16.5838) ccw
  line L8 (6.4367, -16.7547) -> (6.5381, -16.7211)
  line L9 (6.5381, -16.7211) -> (6.6353, -16.677)
  arc A21 (6.6353, -16.677) -> (6.7372, -16.4765) centre (6.561, -16.5131) ccw
  arc A22 (6.7156, -16.1981) -> (6.7372, -16.4765) centre (7.8143, -16.253) ccw
  arc A23 (7.7679, -15.7206) -> (6.7156, -16.1981) centre (7.3648, -16.2305) ccw
  arc A24 (7.9632, -15.9202) -> (7.7679, -15.7206) centre (7.0857, -16.5836) ccw
  arc A25 (7.9632, -15.9202) -> (8.1812, -15.9756) centre (8.1068, -15.8117) ccw
  line L10 (8.1812, -15.9756) -> (8.2784, -15.9315)
  line L11 (8.2784, -15.9315) -> (8.3704, -15.8772)
  arc A26 (8.3704, -15.8772) -> (8.4504, -15.6671) centre (8.279, -15.7222) ccw
  arc A27 (8.3993, -15.3925) -> (8.4504, -15.6671) centre (9.4976, -15.3303) ccw
  arc A28 (9.3949, -14.8059) -> (8.3993, -15.3925) centre (9.0483, -15.3558) ccw
  arc A29 (9.6103, -14.9836) -> (9.3949, -14.8059) centre (8.8083, -15.7364) ccw
  arc A30 (9.6103, -14.9836) -> (9.8329, -15.0155) centre (9.7416, -14.8604) ccw
  line L12 (9.8329, -15.0155) -> (9.9249, -14.9613)
  line L13 (9.9249, -14.9613) -> (10.0106, -14.8976)
  arc A31 (10.0106, -14.8976) -> (10.0678, -14.6801) centre (9.9033, -14.7531) ccw
  arc A32 (9.9879, -14.4125) -> (10.0678, -14.6801) centre (11.0733, -14.2339) ccw
  arc A33 (10.9155, -13.7234) -> (9.9879, -14.4125) centre (10.6293, -14.307) ccw
  arc A34 (11.1485, -13.8772) -> (10.9155, -13.7234) centre (10.4311, -14.711) ccw
  arc A35 (11.1485, -13.8772) -> (11.3733, -13.8852) centre (11.2659, -13.7407) ccw
  line L14 (11.3733, -13.8852) -> (11.459, -13.8215)
  line L15 (11.459, -13.8215) -> (11.5374, -13.7491)
  arc A36 (11.5374, -13.7491) -> (11.5712, -13.5268) centre (11.4153, -13.6169) ccw
  arc A37 (11.4633, -13.2692) -> (11.5712, -13.5268) centre (12.5235, -12.9763) ccw
  arc A38 (12.3123, -12.4854) -> (11.4633, -13.2692) centre (12.0898, -13.0961) ccw
  arc A39 (12.5604, -12.6135) -> (12.3123, -12.4854) centre (11.9357, -13.5189) ccw
  arc A40 (12.5604, -12.6135) -> (12.7848, -12.5977) centre (12.6627, -12.4654) ccw
  line L16 (12.7848, -12.5977) -> (12.8632, -12.5252)
  line L17 (12.8632, -12.5252) -> (12.9335, -12.4449)
  arc A41 (12.9335, -12.4449) -> (12.9434, -12.2202) centre (12.7981, -12.3263) ccw
  arc A42 (12.8087, -11.9756) -> (12.9434, -12.2202) centre (13.8319, -11.5716) ccw
  arc A43 (13.5697, -11.106) -> (12.8087, -11.9756) centre (13.4133, -11.7369) ccw
  arc A44 (13.83, -11.207) -> (13.5697, -11.106) centre (13.3051, -12.1736) ccw
  arc A45 (13.83, -11.207) -> (14.0514, -11.1673) centre (13.9159, -11.0488) ccw
  line L18 (14.0514, -11.1673) -> (14.1217, -11.087)
  line L19 (14.1217, -11.087) -> (14.1831, -10.9996)
  arc A46 (14.1831, -10.9996) -> (14.169, -10.7752) centre (14.0358, -10.8962) ccw
  arc A47 (14.0091, -10.5463) -> (14.169, -10.7752) centre (14.9835, -10.0358) ccw
  arc A48 (14.6733, -9.6007) -> (14.0091, -10.5463) centre (14.5849, -10.2446) ccw
  arc A49 (14.9429, -9.6735) -> (14.6733, -9.6007) centre (14.5237, -10.6904) ccw
  arc A50 (14.9429, -9.6735) -> (15.1588, -9.6105) centre (15.0115, -9.507) ccw
  line L20 (15.1588, -9.6105) -> (15.2202, -9.5231)
  line L21 (15.2202, -9.5231) -> (15.2719, -9.4297)
  arc A51 (15.2719, -9.4297) -> (15.2341, -9.208) centre (15.1144, -9.3425) ccw
  arc A52 (15.0507, -8.9974) -> (15.2341, -9.208) centre (15.9653, -8.3863) ccw
  arc A53 (15.6107, -7.9866) -> (15.0507, -8.9974) centre (15.5912, -8.6363) ccw
  arc A54 (15.8865, -8.0303) -> (15.6107, -7.9866) centre (15.5777, -9.0861) ccw
  arc A55 (15.8865, -8.0303) -> (16.0944, -7.9448) centre (15.937, -7.8576) ccw
  line L22 (16.0944, -7.9448) -> (16.1462, -7.8514)
  line L23 (16.1462, -7.8514) -> (16.1877, -7.753)
  arc A56 (16.1877, -7.753) -> (16.1266, -7.5366) centre (16.0219, -7.683) ccw
  arc A57 (15.9218, -7.3467) -> (16.1266, -7.5366) centre (16.7663, -6.6418) ccw
  arc A58 (16.3712, -6.282) -> (15.9218, -7.3467) centre (16.4208, -6.9301) ccw
  arc A59 (16.65, -6.2962) -> (16.3712, -6.282) centre (16.4552, -7.3788) ccw
  arc A60 (16.65, -6.2962) -> (16.8477, -6.189) centre (16.6819, -6.1191) ccw
  line L24 (16.8477, -6.189) -> (16.8893, -6.0907)
  line L25 (16.8893, -6.0907) -> (16.9201, -5.9884)
  arc A61 (16.9201, -5.9884) -> (16.8363, -5.7798) centre (16.7478, -5.9365) ccw
  arc A62 (16.6125, -5.6127) -> (16.8363, -5.7798) centre (17.3773, -4.822) ccw
  arc A63 (16.9461, -4.5063) -> (16.6125, -5.6127) centre (17.0644, -5.1455) ccw
  arc A64 (17.225, -4.4907) -> (16.9461, -4.5063) centre (17.1463, -5.5879) ccw
  arc A65 (17.225, -4.4907) -> (17.4102, -4.3632) centre (17.2378, -4.3112) ccw
  line L26 (17.4102, -4.3632) -> (17.441, -4.2609)
  line L27 (17.441, -4.2609) -> (17.4608, -4.156)
  arc A66 (17.4608, -4.156) -> (17.3553, -3.9574) centre (17.2839, -4.1227) ccw
  arc A67 (17.115, -3.8151) -> (17.3553, -3.9574) centre (17.7914, -2.9476) ccw
  arc A68 (17.3291, -2.6795) -> (17.115, -3.8151) centre (17.5147, -3.3025) ccw
  arc A69 (17.6047, -2.6344) -> (17.3291, -2.6795) centre (17.6432, -3.7337) ccw
  arc A70 (17.6047, -2.6344) -> (17.7753, -2.4879) centre (17.5984, -2.4545) ccw
  line L28 (17.7753, -2.4879) -> (17.7951, -2.3829)
  line L29 (17.7951, -2.3829) -> (17.8036, -2.2765)
  arc A71 (17.8036, -2.2765) -> (17.6776, -2.0903) centre (17.6242, -2.2622) ccw
  arc A72 (17.4236, -1.9742) -> (17.6776, -2.0903) centre (18.0039, -1.0398) ccw
  arc A73 (17.5158, -0.8224) -> (17.4236, -1.9742) centre (17.7665, -1.4221) ccw
  arc A74 (17.785, -0.7482) -> (17.5158, -0.8224) centre (17.9401, -1.8372) ccw
  arc A75 (17.785, -0.7482) -> (17.939, -0.5844) centre (17.7596, -0.57) ccw
  line L30 (17.939, -0.5844) -> (17.9476, -0.4779)
  line L31 (17.9476, -0.4779) -> (17.9447, -0.3712)
  arc A76 (17.9447, -0.3712) -> (17.7996, -0.1994) centre (17.7648, -0.376) ccw
  arc A77 (17.5347, -0.111) -> (17.7996, -0.1994) centre (18.0124, 0.8798) ccw
  arc A78 (17.504, 1.0441) -> (17.5347, -0.111) centre (17.817, 0.4745) ccw
  arc A79 (17.7638, 1.1465) -> (17.504, 1.0441) centre (18.0337, 0.0801) ccw
  arc A80 (17.7638, 1.1465) -> (17.8995, 1.3257) centre (17.7196, 1.3209) ccw
  line L32 (17.8995, 1.3257) -> (17.8967, 1.4325)
  line L33 (17.8967, 1.4325) -> (17.8825, 1.5383)
  arc A81 (17.8825, 1.5383) -> (17.72, 1.6937) centre (17.7041, 1.5144) ccw
  arc A82 (17.4472, 1.7534) -> (17.72, 1.6937) centre (17.8169, 2.7894) ccw
  arc A83 (17.2938, 2.8988) -> (17.4472, 1.7534) centre (17.6656, 2.3656) ccw
  arc A84 (17.5413, 3.0281) -> (17.2938, 2.8988) centre (17.9231, 1.9965) ccw
  arc A85 (17.5413, 3.0281) -> (17.6572, 3.2208) centre (17.4788, 3.1969) ccw
  line L34 (17.6572, 3.2208) -> (17.643, 3.3267)
  line L35 (17.643, 3.3267) -> (17.6177, 3.4304)
  arc A86 (17.6177, 3.4304) -> (17.4396, 3.5676) centre (17.4428, 3.3877) ccw
  arc A87 (17.162, 3.598) -> (17.4396, 3.5676) centre (17.4194, 4.6674) ccw
  arc A88 (16.8877, 4.7206) -> (17.162, 3.598) centre (17.3141, 4.23) ccw
  arc A89 (17.12, 4.8755) -> (16.8877, 4.7206) centre (17.6093, 3.8903) ccw
  arc A90 (17.12, 4.8755) -> (17.2148, 5.0794) centre (17.04, 5.0367) ccw
  line L36 (17.2148, 5.0794) -> (17.1895, 5.1832)
  line L37 (17.1895, 5.1832) -> (17.1533, 5.2836)
  arc A91 (17.1533, 5.2836) -> (16.9615, 5.4011) centre (16.9839, 5.2225) ccw
  arc A92 (16.6823, 5.4018) -> (16.9615, 5.4011) centre (16.8246, 6.4926) ccw
  arc A93 (16.2903, 6.4889) -> (16.6823, 5.4018) centre (16.7664, 6.0464) ccw
  arc A94 (16.5048, 6.6676) -> (16.2903, 6.4889) centre (17.096, 5.74) ccw
  arc A95 (16.5048, 6.6676) -> (16.5774, 6.8805) centre (16.4081, 6.8194) ccw
  line L38 (16.5774, 6.8805) -> (16.5412, 6.9809)
  line L39 (16.5412, 6.9809) -> (16.4945, 7.0769)
  arc A96 (16.4945, 7.0769) -> (16.2913, 7.1734) centre (16.3326, 6.9982) ccw
  arc A97 (16.0136, 7.1444) -> (16.2913, 7.1734) centre (16.0392, 8.2441) ccw
  arc A98 (15.5083, 8.1837) -> (16.0136, 7.1444) centre (16.0287, 7.7943) ccw
  arc A99 (15.7026, 8.3842) -> (15.5083, 8.1837) centre (16.3891, 7.5247) ccw
  arc A100 (15.7026, 8.3842) -> (15.7521, 8.6036) centre (15.5902, 8.5249) ccw
  line L40 (15.7521, 8.6036) -> (15.7054, 8.6996)
  line L41 (15.7054, 8.6996) -> (15.6488, 8.7901)
  arc A101 (15.6488, 8.7901) -> (15.4366, 8.8645) centre (15.4962, 8.6946) ccw
  arc A102 (15.1635, 8.8061) -> (15.4366, 8.8645) centre (15.072, 9.9023) ccw
  arc A103 (14.5505, 9.7857) -> (15.1635, 8.8061) centre (15.1094, 9.4539) ccw
  arc A104 (14.7224, 10.0058) -> (14.5505, 9.7857) centre (15.4964, 9.2241) ccw
  arc A105 (14.7224, 10.0058) -> (14.7484, 10.2292) centre (14.5958, 10.1337) ccw
  line L42 (14.7484, 10.2292) -> (14.6917, 10.3197)
  line L43 (14.6917, 10.3197) -> (14.6258, 10.4037)
  arc A106 (14.6258, 10.4037) -> (14.4069, 10.455) centre (14.4842, 10.2925) ccw
  arc A107 (14.1415, 10.368) -> (14.4069, 10.455) centre (13.9341, 11.4483) ccw
  arc A108 (13.428, 11.2769) -> (14.1415, 10.368) centre (14.019, 11.0063) ccw
  arc A109 (13.5755, 11.514) -> (13.428, 11.2769) centre (14.4281, 10.819) ccw
  arc A110 (13.5755, 11.514) -> (13.5775, 11.7389) centre (13.436, 11.6277) ccw
  line L44 (13.5775, 11.7389) -> (13.5116, 11.8229)
  line L45 (13.5116, 11.8229) -> (13.4371, 11.8994)
  arc A111 (13.4371, 11.8994) -> (13.214, 11.9272) centre (13.3082, 11.7738) ccw
  arc A112 (12.9594, 11.8124) -> (13.214, 11.9272) centre (12.6383, 12.8645) ccw
  arc A113 (12.1532, 12.6403) -> (12.9594, 11.8124) centre (12.7696, 12.4341) ccw
  arc A114 (12.2747, 12.8918) -> (12.1532, 12.6403) centre (13.1964, 12.2914) ccw
  arc A115 (12.2747, 12.8918) -> (12.2528, 13.1156) centre (12.1239, 12.99) ccw
  line L46 (12.2528, 13.1156) -> (12.1784, 13.1921)
  line L47 (12.1784, 13.1921) -> (12.0962, 13.2602)
  arc A116 (12.0962, 13.2602) -> (11.8713, 13.2642) centre (11.9813, 13.1217) ccw
  arc A117 (11.6304, 13.123) -> (11.8713, 13.2642) centre (11.1993, 14.135) ccw
  arc A118 (10.7408, 13.8605) -> (11.6304, 13.123) centre (11.3756, 13.721) ccw
  arc A119 (10.8349, 14.1234) -> (10.7408, 13.8605) centre (11.8151, 13.6244) ccw
  arc A120 (10.8349, 14.1234) -> (10.7893, 14.3437) centre (10.6744, 14.2051) ccw
  line L48 (10.7893, 14.3437) -> (10.7071, 14.4118)
  line L49 (10.7071, 14.4118) -> (10.6182, 14.4708)
  arc A121 (10.6182, 14.4708) -> (10.3942, 14.4509) centre (10.5187, 14.3209) ccw
  arc A122 (10.1696, 14.2849) -> (10.3942, 14.4509) centre (9.6334, 15.2453) ccw
  arc A123 (9.2067, 14.9237) -> (10.1696, 14.2849) centre (9.8527, 14.8524) ccw
  arc A124 (9.2722, 15.1951) -> (9.2067, 14.9237) centre (10.3, 14.8031) ccw
  arc A125 (9.2722, 15.1951) -> (9.2036, 15.4093) centre (9.1041, 15.2593) ccw
  line L50 (9.2036, 15.4093) -> (9.1146, 15.4683)
  line L51 (9.1146, 15.4683) -> (9.0199, 15.5175)
  arc A126 (9.0199, 15.5175) -> (8.7992, 15.4738) centre (8.9369, 15.3578) ccw
  arc A127 (8.5936, 15.2849) -> (8.7992, 15.4738) centre (7.9583, 16.1829) ccw
  arc A128 (7.5682, 15.8177) -> (8.5936, 15.2849) centre (8.2182, 15.8156) ccw
  arc A129 (7.6046, 16.0946) -> (7.5682, 15.8177) centre (8.6682, 15.8141) ccw
  arc A130 (7.6046, 16.0946) -> (7.5135, 16.3002) centre (7.4305, 16.1405) ccw
  line L52 (7.5135, 16.3002) -> (7.4188, 16.3495)
  line L53 (7.4188, 16.3495) -> (7.3193, 16.3884)
  arc A131 (7.3193, 16.3884) -> (7.1046, 16.3215) centre (7.2538, 16.2207) ccw
  arc A132 (6.9202, 16.1118) -> (7.1046, 16.3215) centre (6.1931, 16.9372) ccw
  arc A133 (5.844, 16.5326) -> (6.9202, 16.1118) centre (6.4906, 16.5995) ccw
  arc A134 (5.8507, 16.8117) -> (5.844, 16.5326) centre (6.9382, 16.6458) ccw
  arc A135 (5.8507, 16.8117) -> (5.7384, 17.0065) centre (5.6728, 16.8389) ccw
  line L54 (5.7384, 17.0065) -> (5.6389, 17.0454)
  line L55 (5.6389, 17.0454) -> (5.5359, 17.0735)
  arc A136 (5.5359, 17.0735) -> (5.3295, 16.9842) centre (5.4885, 16.8998) ccw
  arc A137 (5.1684, 16.7561) -> (5.3295, 16.9842) centre (4.3577, 17.4995) ccw
  arc A138 (4.0536, 17.0601) -> (5.1684, 16.7561) centre (4.6894, 17.1954) ccw
  arc A139 (4.0306, 17.3384) -> (4.0536, 17.0601) centre (5.1295, 17.289) ccw
  arc A140 (4.0306, 17.3384) -> (3.8982, 17.5201) centre (3.8508, 17.3465) ccw
  line L56 (3.8982, 17.5201) -> (3.7951, 17.5482)
  line L57 (3.7951, 17.5482) -> (3.6897, 17.5652)
  arc A141 (3.6897, 17.5652) -> (3.494, 17.4544) centre (3.6611, 17.3875) ccw
  arc A142 (3.3581, 17.2105) -> (3.494, 17.4544) centre (2.4729, 17.8636) ccw
  arc A143 (2.2173, 17.3943) -> (3.3581, 17.2105) centre (2.835, 17.5964) ccw
  arc A144 (2.1648, 17.6686) -> (2.2173, 17.3943) centre (3.2627, 17.7363) ccw
  arc A145 (2.1648, 17.6686) -> (2.0138, 17.8352) centre (1.9852, 17.6575) ccw
  line L58 (2.0138, 17.8352) -> (1.9084, 17.8522)
  line L59 (1.9084, 17.8522) -> (1.8018, 17.8579)
  arc A146 (1.8018, 17.8579) -> (1.6189, 17.727) centre (1.7922, 17.6782) ccw
  arc A147 (1.5097, 17.47) -> (1.6189, 17.727) centre (0.5601, 18.0252) ccw
  arc A148 (0.3558, 17.5315) -> (1.5097, 17.47) centre (0.9486, 17.7981) ccw
  arc A149 (0.2745, 17.7986) -> (0.3558, 17.5315) centre (1.359, 17.9826) ccw
  arc A150 (0.2745, 17.7986) -> (0.1066, 17.9482) centre (0.097, 17.7685) ccw
  line L60 (0.1066, 17.9482) -> (0, 17.9539)
  line L61 (0, 17.9539) -> (-0.1066, 17.9482)
  arc A151 (-0.1066, 17.9482) -> (-0.2745, 17.7986) centre (-0.097, 17.7685) ccw
  arc A152 (-0.3558, 17.5315) -> (-0.2745, 17.7986) centre (-1.359, 17.9826) ccw
  arc A153 (-1.5097, 17.47) -> (-0.3558, 17.5315) centre (-0.9486, 17.7981) ccw
  arc A154 (-1.6189, 17.727) -> (-1.5097, 17.47) centre (-0.5601, 18.0252) ccw
  arc A155 (-1.6189, 17.727) -> (-1.8018, 17.8579) centre (-1.7922, 17.6782) ccw
  line L62 (-1.8018, 17.8579) -> (-1.9084, 17.8522)
  line L63 (-1.9084, 17.8522) -> (-2.0138, 17.8352)
  arc A156 (-2.0138, 17.8352) -> (-2.1648, 17.6686) centre (-1.9852, 17.6575) ccw
  arc A157 (-2.2173, 17.3943) -> (-2.1648, 17.6686) centre (-3.2627, 17.7363) ccw
  arc A158 (-3.3581, 17.2105) -> (-2.2173, 17.3943) centre (-2.835, 17.5964) ccw
  arc A159 (-3.494, 17.4544) -> (-3.3581, 17.2105) centre (-2.4729, 17.8636) ccw
  arc A160 (-3.494, 17.4544) -> (-3.6897, 17.5652) centre (-3.6611, 17.3875) ccw
  line L64 (-3.6897, 17.5652) -> (-3.7951, 17.5482)
  line L65 (-3.7951, 17.5482) -> (-3.8982, 17.5201)
  arc A161 (-3.8982, 17.5201) -> (-4.0306, 17.3384) centre (-3.8508, 17.3465) ccw
  arc A162 (-4.0536, 17.0601) -> (-4.0306, 17.3384) centre (-5.1295, 17.289) ccw
  arc A163 (-5.1684, 16.7561) -> (-4.0536, 17.0601) centre (-4.6894, 17.1954) ccw
  arc A164 (-5.3295, 16.9842) -> (-5.1684, 16.7561) centre (-4.3577, 17.4995) ccw
  arc A165 (-5.3295, 16.9842) -> (-5.5359, 17.0735) centre (-5.4885, 16.8998) ccw
  line L66 (-5.5359, 17.0735) -> (-5.6389, 17.0454)
  line L67 (-5.6389, 17.0454) -> (-5.7384, 17.0065)
  arc A166 (-5.7384, 17.0065) -> (-5.8507, 16.8117) centre (-5.6728, 16.8389) ccw
  arc A167 (-5.844, 16.5326) -> (-5.8507, 16.8117) centre (-6.9382, 16.6458) ccw
  arc A168 (-6.9202, 16.1118) -> (-5.844, 16.5326) centre (-6.4906, 16.5995) ccw
  arc A169 (-7.1046, 16.3215) -> (-6.9202, 16.1118) centre (-6.1931, 16.9372) ccw
  arc A170 (-7.1046, 16.3215) -> (-7.3193, 16.3884) centre (-7.2538, 16.2207) ccw
  line L68 (-7.3193, 16.3884) -> (-7.4188, 16.3495)
  line L69 (-7.4188, 16.3495) -> (-7.5135, 16.3002)